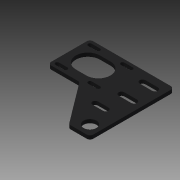
# Autodesk Inventor part: z_motor_mount_plate
Saved by Autodesk Inventor 2013 SP2 (Build 170200200, 200)
## iProperties
Created: 2013-03-06
Part Number: z_motor_mount_plate
Material: Generic
Document SubType Name: Modeling
Designer: Edward
Density: 1 g/cm^3
Description: Z-axis Mounting plate (nema17 style)
Mass: 11.5889 g
Surface Area: 90.4625 cm^2
Volume: 11.5889 cm^3
Vendor: custom
Stock Number: SM_Z1
Author: Edward
Autodesk Inventor part; units mm, degrees
ref_plane "YZ Plane" through (0, 0, 0) normal (1, 0, 0) x (0, 1, 0)
ref_plane "XZ Plane" through (0, 0, 0) normal (0, 1, 0) x (-1, 0, 0)
ref_plane "XY Plane" through (0, 0, 0) normal (0, 0, 1) x (1, 0, 0)
sketch "Sketch1" plane through (0, 0, 0) normal (0, 1, 0) x (-1, 0, 0)
  line L0 (-40, 40) -> (40, 40)
  line L1 (40, 40) -> (40, -40)
  line L2 (40, -40) -> (-40, -40)
  line L3 (-40, -40) -> (-40, 40)
  point P0 (0, 0)
  dimension "d0" = 80
  dimension "d1" = 80
  dimension "d2" = 40
  dimension "d3" = 40
  constraints: 8 end point, 2 parallel, 1 horizontal, 1 perpendicular
  measures "d0" distance of L1.end L2.end
  measures "d1" distance of L0.end L1.end
  measures "d2" distance from line of point (0, 0) L3
  measures "d3" distance from line of L0 point (0, 0)
extrude "Extrusion1" add sketch "Sketch1" along normal blind 3.4163
sketch "Sketch2" plane through (0, 3.4163, 0) normal (0, 1, 0) x (1, 0, 0)
  line L0 (40, -40) -> (40, 40) projected
  line L1 (40, 40) -> (-40, 40) projected
  arc A0 (20, 32.75) -> (20, 27.25) centre (20, 30) ccw
  arc A1 (20, 12.75) -> (20, 7.25) centre (20, 10) ccw
  line L2 (20, 32.75) -> (32, 32.75)
  line L3 (20, 27.25) -> (32, 27.25)
  line L4 (20, 12.75) -> (32, 12.75)
  line L5 (20, 7.25) -> (32, 7.25)
  arc A2 (32, 27.25) -> (32, 32.75) centre (32, 30) ccw
  arc A3 (32, 7.25) -> (32, 12.75) centre (32, 10) ccw
  point P0 (0, 0)
  point P1 (40, 32.75)
  point P2 (40, 27.25)
  point P3 (40, 12.75)
  point P4 (40, 7.25)
  dimension "d6" = 5.5
  dimension "d7" = 5.5
  dimension "d8" = 20
  dimension "d9" = 10
  dimension "d10" = 20
  dimension "d11" = 20
  dimension "d72" = 5.5
  dimension "d73" = 10
  dimension "d74" = 8
  dimension "d75" = 5.5
  dimension "d76" = 20
  dimension "d77" = 8
  constraints: 8 end point, 8 point on circle, 4 centre point, 4 perpendicular, 4 point on line, 4 tangent
  measures "d6" diameter of A0
  measures "d7" diameter of A1
  measures "d8" distance of A0.centre A1.centre
  measures "d9" distance from line of L1 A0.centre
  measures "d10" distance from line of L0 A0.centre
  measures "d11" distance from line of L0 A1.centre
  measures "d72" diameter of A2
  measures "d73" distance from line of L1 A2.centre
  measures "d74" distance from line of L0 A2.centre
  measures "d75" diameter of A3
  measures "d76" distance of A2.centre A3.centre
  measures "d77" distance from line of L0 A3.centre
extrude "Extrusion2" cut sketch "Sketch2" against normal through all
sketch "Sketch3" plane through (0, 3.4163, 0) normal (0, 1, 0) x (1, 0, 0)
  line L0 (40, 40) -> (-40, 40) projected
  line L1 (40, -40) -> (40, 40) projected
  circle A0 centre (30, -30) radius 6.125
  point P0 (40, 7.25)
  point P1 (0, 0)
  dimension "d14" = 12.25
  dimension "d15" = 10
  dimension "d16" = 70
  constraints: 1 centre point
  measures "d14" diameter of A0
  measures "d15" distance from line of L1 A0.centre
  measures "d16" distance from line of L0 A0.centre
extrude "Extrusion3" cut sketch "Sketch3" against normal through all
sketch "Sketch4" plane through (0, 3.4163, 0) normal (0, 1, 0) x (1, 0, 0)
  line L0 (40, 40) -> (-40, 40) projected
  line L1 (-40, 40) -> (-40, -40) projected
  line L2 (-40, -40) -> (40, -40) projected
  line L3 (32, 27.25) -> (20, 27.25) projected
  line L4 (-40, 0) -> (-10, 0)
  line L5 (-10, 0) -> (20, -40)
  point P0 (40, 27.25)
  point P1 (0, 0)
  dimension "d19" = 30
  dimension "d21" = 40
  dimension "d22" = 60
  constraints: 4 end point, 1 midpoint, 1 parallel, 1 point on line
  measures "d19" distance of L4.start L4.end
  measures "d21" distance between parallel lines of L0 L4
  measures "d22" distance from line of L1 L5.end
extrude "Extrusion4" cut sketch "Sketch4" against normal through all
fillet "Fillet1" radius 3 6 edges at (40, 1.7082, 40) (20, 1.7082, 40) (40, 1.7082, -40) (-10, 1.7082, 0) (-40, 1.7082, 0) (-40, 1.7082, -40)
sketch "Sketch5" plane through (0, 3.4163, 0) normal (0, 1, 0) x (1, 0, 0)
  line L0 (40, -37) -> (40, 37) projected
  line L1 (37, 40) -> (-37, 40) projected
  arc A0 (-12, 8.5) -> (-12, 31.5) centre (-12, 20) ccw
  line L2 (-12, 31.5) -> (-22, 31.5)
  line L3 (-12, 8.5) -> (-22, 8.5)
  arc A1 (-22, 31.5) -> (-22, 8.5) centre (-22, 20) ccw
  point P0 (40, 15.75)
  point P1 (40, 24.25)
  point P2 (0, 0)
  dimension "d26" = 23
  dimension "d27" = 52
  dimension "d35" = 23
  dimension "d36" = 10
  dimension "d37" = 10
  dimension "d38" = 20
  dimension "d39" = 20
  dimension "d42" = 52
  dimension "d81" = 8.5
  dimension "d82" = 8.5
  constraints: 4 end point, 4 point on circle, 2 centre point
  measures "d26" diameter of A0
  measures "d27" distance from line of L0 A0.centre
  measures "d35" diameter of A1
  measures "d36" distance of L2.start L2.end
  measures "d37" distance of L3.start L3.end
  measures "d38" distance from line of L1 A0.centre
  measures "d39" distance from line of L1 A1.centre
  measures "d42" distance from line of L0 L3.start
  measures "d81" distance from line of L1 L2.start
  measures "d82" distance from line of L1 L2.end
extrude "Extrusion5" cut sketch "Sketch5" against normal through all
sketch "Sketch6" plane through (0, 3.4163, 0) normal (0, 1, 0) x (1, 0, 0)
  line L0 (40, -37) -> (40, 37) projected
  line L1 (37, 40) -> (-37, 40) projected
  arc A0 (3.5, 33.75) -> (3.5, 37.25) centre (3.5, 35.5) ccw
  arc A1 (-4.5, 37.25) -> (-4.5, 33.75) centre (-4.5, 35.5) ccw
  line L2 (-4.5, 37.25) -> (3.5, 37.25)
  line L3 (3.5, 33.75) -> (-4.5, 33.75)
  point P0 (40, 35.75)
  point P1 (0, 0)
  dimension "d48" = 3.5
  dimension "d49" = 4.5
  dimension "d50" = 36.5
  dimension "d51" = 3.5
  dimension "d52" = 4.5
  dimension "d53" = 44.5
  dimension "d78" = 8
  constraints: 4 end point, 4 point on circle, 3 tangent, 2 centre point
  measures "d48" diameter of A0
  measures "d49" distance from line of L1 A0.centre
  measures "d50" distance from line of L0 A0.centre
  measures "d51" diameter of A1
  measures "d52" distance from line of L1 A1.centre
  measures "d53" distance from line of L0 A1.centre
  measures "d78" distance of L3.start L3.end
extrude "Extrusion6" cut sketch "Sketch6" against normal through all
pattern_linear "Rectangular Pattern1" count 2 spacing 31.1 along (-1, 0, 0) count 2 spacing 31.1 along (0, 0, 1) of "Extrusion6"
sketch "Sketch7" plane through (0, 3.4163, 0) normal (0, 1, 0) x (1, 0, 0)
  line L0 (21.5, -40) -> (37, -40) projected
  line L1 (40, -37) -> (40, 37) projected
  arc A0 (25, -12.625) -> (25, -7.375) centre (25, -10) ccw
  arc A1 (15, -7.375) -> (15, -12.625) centre (15, -10) ccw
  line L2 (15, -7.375) -> (25, -7.375)
  line L3 (25, -12.625) -> (15, -12.625)
  point P0 (40, 4.25)
  point P1 (0, 0)
  dimension "d63" = 5.25
  dimension "d64" = 15
  dimension "d65" = 30
  dimension "d66" = 5.25
  dimension "d67" = 10
  dimension "d68" = 30
  dimension "d69" = 10
  constraints: 4 end point, 4 point on circle, 3 tangent, 2 centre point
  measures "d63" diameter of A0
  measures "d64" distance from line of L1 A0.centre
  measures "d65" distance from line of L0 A0.centre
  measures "d66" diameter of A1
  measures "d67" distance of A0.centre A1.centre
  measures "d68" distance from line of L0 A1.centre
  measures "d69" distance of L3.start L3.end
extrude "Extrusion7" cut sketch "Sketch7" against normal through all
equation "\"d73\" = d9"
equation "\"d76\" = d8"
equation "\"d77\" = d74"
equation "\"d35\" = d26"
equation "\"d42\" = d27"
equation "\"d66\" = d63"
body "Solid1"
